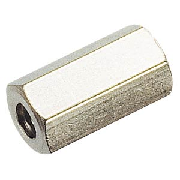
# Autodesk Inventor part: Distanzhuelse_M3x20mm_
Saved by Autodesk Inventor 2016 (Build 200138000, 138)
## iProperties
Created: 2015-10-04
Part Number: Distanzhuelse_M3x20mm_
Material: Nickel-Kupfer-Legierung 400
Document SubType Name: Modeling
Designer: 4ndreas
Density: 8.83 g/cm^3
Appearance: Chrom - poliert
Mass: 3.49173 g
Surface Area: 5.21893 cm^2
Volume: 0.395439 cm^3
Author: 4ndreas
Autodesk Inventor part; units mm, degrees
ref_plane "YZ Plane" through (0, 0, 0) normal (1, 0, 0) x (0, 1, 0)
ref_plane "XZ Plane" through (0, 0, 0) normal (0, 1, 0) x (-1, 0, 0)
ref_plane "XY Plane" through (0, 0, 0) normal (0, 0, 1) x (1, 0, 0)
sketch "Skizze1" plane through (0, 0, 0) normal (0, 0, 1) x (1, 0, 0)
  line L0 (0, 2.8868) -> (2.5, 1.4434)
  line L1 (2.5, 1.4434) -> (2.5, -1.4434)
  line L2 (2.5, -1.4434) -> (0, -2.8868)
  line L3 (0, -2.8868) -> (-2.5, -1.4434)
  line L4 (-2.5, -1.4434) -> (-2.5, 1.4434)
  line L5 (-2.5, 1.4434) -> (0, 2.8868)
  circle A0 centre (0, 0) radius 1.5
  dimension "d0" = 5
  dimension "d1" = 3
  constraints: 12 end point, 2 coincident, 1 centre point, 1 vertical, 13 other
  measures "d0" distance between parallel lines of L4 L1
  measures "d1" diameter of A0
extrude "Extrusion1" add sketch "Skizze1" along normal blind 20
chamfer "Fase1" distance 0.3 angle 45 13 edges at (1.25, -2.1651, 20) (-1.25, -2.1651, 20) (2.5, 0, 20) (1.25, 2.1651, 20) (-1.25, 2.1651, 20) (1.25, -2.1651, 0) (2.5, 0, 0) (-1.25, -2.1651, 0) (1.25, 2.1651, 0) (-1.25, 2.1651, 0) (-2.5, 0, 0) (-1.5, 0, 20) (-1.5, 0, 0)
thread "Gewinde1" size "M3x0.5" class "6H" standard "ANSI Metric M Profile" full length
sketch "Skizze2" plane through (0, 0, 20) normal (0, 0, 1) x (1, 0, 0)
  line L0 (0, -2.5403) -> (-2.5, -1.097) projected
  line L1 (2.2, -1.2702) -> (0, -2.5403) projected
  line L2 (2.2, 1.2702) -> (2.2, -1.2702) projected
  line L3 (0, 2.5403) -> (2.2, 1.2702) projected
  line L4 (-2.5, 1.097) -> (0, 2.5403) projected
  line L5 (-2.5, 1.097) -> (-2.5, -1.097) projected
  circle A0 centre (0, 0) radius 1.8 projected
extrude "Extrusion2" add sketch "Skizze2" against normal blind 10 contours A0
sketch "Skizze3" plane through (0, 0, 20) normal (0, 0, 1) x (1, 0, 0)
  circle A0 centre (0, 0) radius 1.5
  dimension "d11" = 3
  constraints: 1 centre point, 1 coincident
  measures "d11" diameter of A0
extrude "Extrusion3" add sketch "Skizze3" along normal blind 5
thread "Gewinde2" size "M3x0.5" class "6g" standard "ANSI Metric M Profile" full length
chamfer "Fase2" distance 0.3 angle 45 1 edges at (-1.5, 0, 25)
